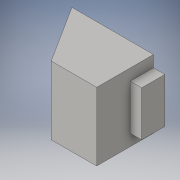
# Autodesk Inventor part: mcdave_summo_robot
Saved by Autodesk Inventor 2016 (Build 200138000, 138)
## iProperties
Created: 2017-08-30
Part Number: mcdave_summo_robot
Material: Generic
Document SubType Name: Modeling
Designer: student
Density: 1 g/cm^3
Appearance: Default
Author: student
Autodesk Inventor part; units mm, degrees
ref_plane "YZ Plane" through (0, 0, 0) normal (1, 0, 0) x (0, 1, 0)
ref_plane "XZ Plane" through (0, 0, 0) normal (0, 1, 0) x (-1, 0, 0)
ref_plane "XY Plane" through (0, 0, 0) normal (0, 0, 1) x (1, 0, 0)
sketch "Sketch1" plane through (0, 0, 0) normal (0, 0, 1) x (1, 0, 0)
  line L0 (40.3102, 67.1309) -> (91.1102, 67.1309)
  line L1 (91.1102, 67.1309) -> (91.1102, -9.0691)
  line L2 (91.1102, -9.0691) -> (40.3102, -9.0691)
  line L3 (40.3102, -9.0691) -> (40.3102, 67.1309)
  point P0 (0, 0)
  dimension "d0" = 50.8
  dimension "d1" = 76.2
  constraints: 8 end point, 2 parallel, 1 horizontal, 1 perpendicular
  measures "d0" distance of L1.end L2.end
  measures "d1" distance of L0.end L1.end
extrude "Extrusion1" add sketch "Sketch1" along normal blind 63.5
sketch "Sketch2" plane through (40.3102, -9.0691, 0) normal (0, -1, 0) x (1, 0, 0)
  line L0 (0, 0) -> (0, 63.5) projected
  line L1 (50.8, 63.5) -> (0, 63.5) projected
  line L2 (0, 0) -> (50.8, 0) projected
  line L3 (0, 0) -> (-40.3102, 0)
  line L4 (0, 63.5) -> (-40.3102, 0)
  constraints: 4 end point, 1 horizontal, 1 point on line
extrude "Extrusion2" add sketch "Sketch2" against normal blind 76.2
sketch "Sketch6" plane through (91.1102, -9.0691, 0) normal (1, 0, 0) x (0, 0, -1)
  line L0 (-63.5, 0) -> (-63.5, 76.2) projected
  line L1 (0, 76.2) -> (0, 0) projected
  line L2 (-25.9302, 38.1) -> (-25.9302, 63.2786)
  line L3 (-25.9302, 63.2786) -> (0, 63.2786)
  line L4 (-25.9302, 38.1) -> (-25.9302, 12.9286)
  line L5 (-25.9302, 38.1) -> (-0.7588, 38.1) construction
  line L6 (-25.9302, 12.9286) -> (0, 12.9286)
  point P0 (0, 9.0691)
  dimension "d11" = 25.1714
  dimension "d12" = 90
  dimension "d13" = 50.35
  dimension "d14" = 25.9302
  constraints: 10 end point, 3 perpendicular, 2 point on line, 1 horizontal, 1 vertical
  measures "d11" distance of L2.start L4.end
  measures "d12" angle of L4 L5
  measures "d13" distance of L2.end L4.end
  measures "d14" distance of L2.end L3.end
extrude "Extrusion3" add sketch "Sketch6" along normal blind 12.7
body "Solid1"
